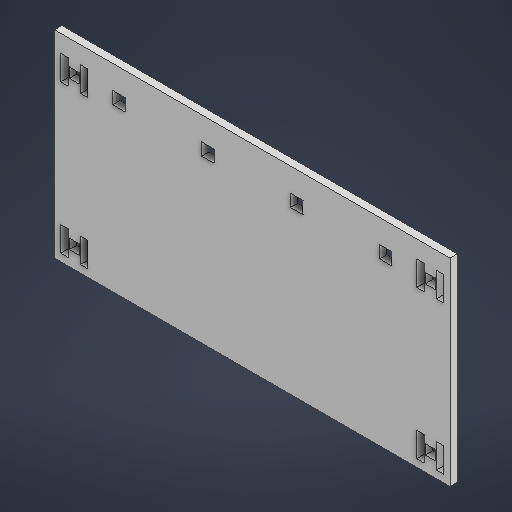
# Autodesk Inventor part: techo
Saved by Autodesk Inventor 2026 (Build 300175000, 175)
## iProperties
Created: 2026-05-15
Part Number: techo
Material: Generic
Document SubType Name: Modeling
Designer: juana
Density: 1 g/cm^3
Appearance: Default
Author: juana
Autodesk Inventor part; units mm, degrees
ref_plane "YZ Plane" through (0, 0, 0) normal (1, 0, 0) x (0, 1, 0)
ref_plane "XZ Plane" through (0, 0, 0) normal (0, 1, 0) x (-1, 0, 0)
ref_plane "XY Plane" through (0, 0, 0) normal (0, 0, 1) x (1, 0, 0)
sketch "Sketch1" plane through (0, 0, 0) normal (0, 0, 1) x (1, 0, 0)
  line L0 (0, 0) -> (160, 0)
  line L1 (160, 0) -> (160, 80)
  line L2 (160, 80) -> (0, 80)
  line L3 (0, 80) -> (0, 0)
  line L4 (2.5, 13) -> (5.5, 13)
  line L5 (5.5, 13) -> (5.5, 3)
  line L6 (5.5, 3) -> (2.5, 3)
  line L7 (2.5, 3) -> (2.5, 13)
  line L8 (10.5, 13) -> (13.5, 13)
  line L9 (13.5, 13) -> (13.5, 3)
  line L10 (13.5, 3) -> (10.5, 3)
  line L11 (10.5, 3) -> (10.5, 13)
  line L12 (0, 40) -> (160, 40) construction
  line L13 (80, 80) -> (80, 0) construction
  line L14 (0, 0) -> (0, 80)
  line L15 (2.5, 77) -> (2.5, 67) construction
  line L16 (13.5, 77) -> (10.5, 77)
  line L17 (157.5, 13) -> (154.5, 13)
  line L18 (154.5, 13) -> (154.5, 3)
  line L19 (154.5, 3) -> (157.5, 3)
  line L20 (157.5, 3) -> (157.5, 13)
  line L21 (149.5, 13) -> (146.5, 13)
  line L22 (146.5, 13) -> (146.5, 3)
  line L23 (146.5, 3) -> (149.5, 3)
  line L24 (149.5, 3) -> (149.5, 13)
  line L25 (2.5, 77) -> (157.5, 77) construction
  line L26 (157.5, 77) -> (157.5, 3) construction
  line L27 (157.5, 3) -> (2.5, 3) construction
  line L28 (2.5, 3) -> (2.5, 77) construction
  line L29 (5.5, 13) -> (5.5, 3)
  line L30 (6, 6) -> (10, 6)
  line L31 (10, 6) -> (10, 10)
  line L32 (10, 10) -> (6, 10)
  line L33 (6, 10) -> (6, 6)
  line L34 (23.49, 65.49) -> (28.51, 65.49)
  line L35 (28.51, 65.49) -> (28.51, 70.51)
  line L36 (28.51, 70.51) -> (23.49, 70.51)
  line L37 (23.49, 70.51) -> (23.49, 65.49)
  line L38 (59.49, 65.49) -> (64.51, 65.49)
  line L39 (64.51, 70.51) -> (59.49, 70.51)
  line L40 (64.51, 65.49) -> (64.51, 70.51)
  line L41 (59.49, 70.51) -> (59.49, 65.49)
  line L42 (95.49, 65.49) -> (100.51, 65.49)
  line L43 (100.51, 70.51) -> (95.49, 70.51)
  line L44 (100.51, 65.49) -> (100.51, 70.51)
  line L45 (95.49, 70.51) -> (95.49, 65.49)
  line L46 (131.49, 65.49) -> (136.51, 65.49)
  line L47 (136.51, 70.51) -> (131.49, 70.51)
  line L48 (136.51, 65.49) -> (136.51, 70.51)
  line L49 (131.49, 70.51) -> (131.49, 65.49)
  line L50 (2.5, 73) -> (5.5, 73)
  line L51 (5.5, 73) -> (5.5, 63)
  line L52 (5.5, 63) -> (2.5, 63)
  line L53 (2.5, 63) -> (2.5, 73)
  line L54 (6, 70) -> (10, 70)
  line L55 (10, 70) -> (10, 66)
  line L56 (10, 66) -> (6, 66)
  line L57 (6, 66) -> (6, 70)
  line L58 (10.5, 73) -> (13.5, 73)
  line L59 (13.5, 73) -> (13.5, 63)
  line L60 (13.5, 63) -> (10.5, 63)
  line L61 (10.5, 63) -> (10.5, 73)
  line L62 (157.5, 77) -> (157.5, 67) construction
  line L63 (157.5, 3) -> (157.5, 77) construction
  line L64 (157.5, 73) -> (154.5, 73)
  line L65 (154.5, 73) -> (154.5, 63)
  line L66 (154.5, 63) -> (157.5, 63)
  line L67 (157.5, 63) -> (157.5, 73)
  line L68 (154, 70) -> (150, 70)
  line L69 (150, 70) -> (150, 66)
  line L70 (150, 66) -> (154, 66)
  line L71 (154, 66) -> (154, 70)
  line L72 (149.5, 73) -> (146.5, 73)
  line L73 (146.5, 73) -> (146.5, 63)
  line L74 (146.5, 63) -> (149.5, 63)
  line L75 (149.5, 63) -> (149.5, 73)
  line L76 (154.5, 13) -> (154.5, 3)
  line L77 (150, 6) -> (150, 10)
  line L78 (150, 10) -> (154, 10)
  line L79 (154, 10) -> (154, 6)
  line L80 (154, 6) -> (150, 6)
  point P0 (23.49, 68)
  point P1 (26, 70.51)
  point P2 (62, 70.51)
  point P3 (59.49, 68)
  point P4 (98, 70.51)
  point P5 (95.49, 68)
  point P6 (134, 70.51)
  point P7 (131.49, 68)
  point P8 (2.5, 72)
  point P9 (5.5, 68)
  point P10 (6, 68)
  point P11 (8, 66)
  point P12 (8, 10)
  point P13 (157.5, 72)
  point P14 (154.5, 68)
  point P15 (154, 68)
  point P16 (152, 66)
  dimension "d0" = 80
  dimension "d1" = 160
  dimension "d2" = 3
  dimension "d3" = 2.5
  dimension "d4" = 3
  dimension "d5" = 10
  dimension "d6" = 5
  dimension "d11" = 5.02
  dimension "d12" = 5.02
  dimension "d13" = 23.5
  dimension "d16" = 36
  dimension "d23" = 70
  dimension "d24" = 3
  dimension "d25" = 3
  dimension "d26" = 0.5
  dimension "d27" = 0.5
  constraints: 162 end point, 36 symmetric about line, 16 parallel, 11 midpoint, 9 horizontal, 8 equal length, 8 perpendicular, 4 horizontal alignment, 3 vertical alignment, 2 point on line, 30 other
  measures "d0" distance of L0.end L1.end
  measures "d1" distance of L0.start L0.end
  measures "d2" distance of L4.start L4.end
  measures "d3" distance between parallel lines of L3 L7
  measures "d4" distance between parallel lines of L0 L6
  measures "d5" distance of L4.end L5.end
  measures "d6" distance between parallel lines of L11 L5
  measures "d11" distance of L35.end L36.end
  measures "d12" distance of L34.end L35.end
  measures "d13" distance from line of L28 point (26, 70.51)
  measures "d16" distance of L34.end L38.end
  measures "d23" distance from line of L6.end L50
  measures "d24" distance between parallel lines of L8 L32
  measures "d25" distance between parallel lines of L27 L30
  measures "d26" distance between parallel lines of L11 L31
  measures "d27" distance between parallel lines of L5 L33
extrude "Extrusion1" add sketch "Sketch1" along normal blind 3
body "Solid1"
